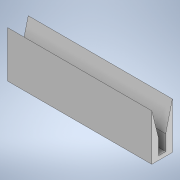
# Autodesk Inventor part: edge holder
Saved by Autodesk Inventor 2021 (Build 250183000, 183)
## iProperties
Created: 2021-06-29
Part Number: edge holder
Material: Generic
Document SubType Name: Modeling
Designer: newic
Density: 1 g/cm^3
Appearance: Default
Author: newic
Autodesk Inventor part; units mm, degrees
ref_plane "YZ Plane" through (0, 0, 0) normal (1, 0, 0) x (0, 1, 0)
ref_plane "XZ Plane" through (0, 0, 0) normal (0, 1, 0) x (-1, 0, 0)
ref_plane "XY Plane" through (0, 0, 0) normal (0, 0, 1) x (1, 0, 0)
sketch "Sketch1" plane through (0, 0, 0) normal (1, 0, 0) x (0, 1, 0)
  line L0 (0, 0) -> (3.175, 0)
  line L1 (3.175, -12.7) -> (0, -12.7)
  line L2 (0, -12.7) -> (0, 0)
  line L3 (3.175, 0) -> (28.575, 0)
  line L4 (3.175, -12.7) -> (28.575, -12.7)
  line L5 (12.065, -4.1275) -> (28.575, 0)
  line L6 (12.065, -8.5725) -> (28.575, -12.7)
  line L7 (12.065, -4.1275) -> (3.175, -4.1275)
  line L8 (12.065, -8.5725) -> (3.175, -8.5725)
  line L9 (3.175, -4.1275) -> (2.54, -4.1275)
  line L10 (2.54, -4.1275) -> (2.54, -8.5725)
  line L11 (2.54, -8.5725) -> (3.175, -8.5725)
  dimension "d0" = 3.175
  dimension "d1" = 12.7
  dimension "d2" = 25.4
  dimension "d5" = 0.635
  constraints: 24 end point, 3 horizontal, 1 parallel, 1 perpendicular, 1 vertical
  measures "d0" distance of L1.start L1.end
  measures "d1" distance of L0.end L1.start
  measures "d2" distance of L0.end L3.end
  measures "d5" distance of L7.end L9.end
extrude "Extrusion1" add sketch "Sketch1" along normal blind 88.9
body "Solid1"
